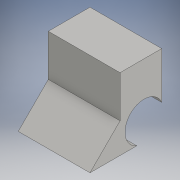
# Autodesk Inventor part: Aidan Sherry Frame
Saved by Autodesk Inventor 2016 (Build 200138000, 138)
## iProperties
Created: 2017-11-13
Part Number: Aidan Sherry Frame
Material: Generic
Document SubType Name: Modeling
Designer: Student
Density: 1 g/cm^3
Appearance: Default
Author: Student
Autodesk Inventor part; units mm, degrees
ref_plane "YZ Plane" through (0, 0, 0) normal (1, 0, 0) x (0, 1, 0)
ref_plane "XZ Plane" through (0, 0, 0) normal (0, 1, 0) x (-1, 0, 0)
ref_plane "XY Plane" through (0, 0, 0) normal (0, 0, 1) x (1, 0, 0)
sketch "Sketch1" plane through (0, 0, 0) normal (0, 0, 1) x (1, 0, 0)
  line L0 (-8.1293, 50) -> (50, 50)
  line L1 (50, 50) -> (50, -14.9785)
  line L2 (-50, -50) -> (-8.1293, -8.1293)
  line L3 (-8.1293, 50) -> (-8.1293, -8.1293)
  arc A0 (50, -14.9785) -> (15.2248, -50) centre (25.4341, -25.3614) ccw
  line L4 (15.2248, -50) -> (-50, -50)
  point P0 (0, 0)
  dimension "d5" = 53.34
  constraints: 10 end point, 2 point on circle, 2 point on line, 1 centre point, 1 horizontal, 1 parallel, 1 vertical
  measures "d5" diameter of A0
extrude "Extrusion1" add sketch "Sketch1" along normal blind 100
body "Solid1"
